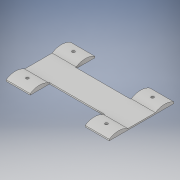
# Autodesk Inventor part: TapeMeasureBracketTop
Saved by Autodesk Inventor 2019 (Build 230136000, 136)
## iProperties
Created: 2018-11-07
Part Number: TapeMeasureBracketTop
Material: Generic
Document SubType Name: Modeling
Designer: Ashley
Density: 1 g/cm^3
Appearance: Default
Author: Ashley
Autodesk Inventor part; units mm, degrees
ref_plane "YZ Plane" through (0, 0, 0) normal (1, 0, 0) x (0, 1, 0)
ref_plane "XZ Plane" through (0, 0, 0) normal (0, 1, 0) x (-1, 0, 0)
ref_plane "XY Plane" through (0, 0, 0) normal (0, 0, 1) x (1, 0, 0)
sketch "Main Base Sketch" plane through (0, 0, 0) normal (0, 1, 0) x (-1, 0, 0)
  line L0 (75, -47) -> (75, 47)
  line L1 (-75, 47) -> (-75, -47)
  line L2 (-75, -47) -> (75, 47) construction
  line L3 (75, -47) -> (-75, 47) construction
  line L4 (-40, -47) -> (-40, -19)
  line L5 (-40, -19) -> (40, -19)
  line L6 (40, -19) -> (40, -47)
  line L7 (40, 19) -> (40, 47)
  line L8 (-40, 19) -> (40, 19)
  line L9 (-40, 47) -> (-40, 19)
  line L10 (75, 47) -> (40, 47)
  line L11 (-40, 47) -> (-75, 47)
  line L12 (-75, -47) -> (-40, -47)
  line L13 (40, -47) -> (75, -47)
  point P0 (0, 0)
  point P1 (0, 0)
  dimension "d0" = 94
  dimension "d1" = 35
  dimension "d2" = 35
  dimension "d3" = 80
  dimension "d4" = 150
  dimension "d5" = 28
  dimension "d6" = 94
  dimension "d8" = 80
  dimension "d9" = 28
  dimension "d27" = 28
  dimension "d28" = 38
  dimension "d37" = 0
  constraints: 28 end point, 6 parallel, 5 perpendicular, 2 horizontal, 2 midpoint
  measures "d0" distance of L0.start L0.end
  measures "d1" distance between parallel lines of L6 L0
  measures "d2" distance between parallel lines of L1 L4
  measures "d3" distance of L4.end L5.end
  measures "d4" distance between parallel lines of L1 L0
  measures "d5" distance of L5.end L6.end
  measures "d6" distance of L1.start L1.end
  measures "d8" distance of L8.start L7.start
  measures "d9" distance of L9.start L8.start
  measures "d27" distance of L7.start L7.end
  measures "d28" distance between parallel lines of L5 L8
  measures "d37" distance of point (0, 0) point (0, 0)
extrude "Main Base Extrusion" add sketch "Main Base Sketch" along normal blind 6
sketch "Middle Cut Sketch" plane through (0, 6, 0) normal (0, 1, 0) x (1, 0, 0)
  line L0 (-75, 47) -> (-75, -47) projected
  line L1 (75, 19) -> (-75, 19)
  line L2 (-75, 19) -> (-75, -19)
  line L3 (-75, -19) -> (75, -19)
  line L4 (75, -19) -> (75, 19)
  line L5 (-40, -19) -> (40, -19) projected
  line L6 (75, -47) -> (75, 47) projected
  line L7 (40, 19) -> (-40, 19) projected
  point P0 (0, 0)
  dimension "d18" = 0
  dimension "d19" = 0
  dimension "d34" = 0
  constraints: 8 end point, 2 parallel, 1 horizontal, 1 perpendicular, 1 point on line
  measures "d18" distance between parallel lines of L5 L3
  measures "d19" distance between parallel lines of L6 L4
  measures "d34" distance between parallel lines of L7 L1
extrude "Middle Cut" cut sketch "Middle Cut Sketch" against normal blind 4
sketch "Arc Sketch" plane through (75, 0, 47) normal (1, 0, 0) x (0, 0, -1)
  line L0 (27, 9.4354) -> (27, -6.3008)
  line L1 (13.5, 8.8022) -> (13.5, -9.7521)
  line L2 (-4.6363, 2) -> (37.5698, 2)
  line L3 (94, 0) -> (0, 0) projected
  arc A0 (27, 2) -> (0, 2) centre (13.5, -18.7813) ccw
  line L4 (0, 7.9962) -> (0, -1.9448)
  line L5 (0, 0) -> (0, 6) projected
  line L6 (0, 6) -> (0, 2)
  line L7 (28, 6) -> (0, 6) projected
  line L8 (0, 6) -> (28, 6)
  line L9 (28, 2) -> (28, 6) projected
  line L10 (28, 6) -> (28, 2)
  line L11 (28, 2) -> (27, 2)
  line L12 (94, 0) -> (94, 6) projected
  dimension "d25" = 13.5
  dimension "d26" = 2
  dimension "d29" = 13.5
  dimension "d30" = 27
  constraints: 16 end point, 3 point on line, 3 vertical, 2 collinear, 2 point on circle, 1 centre point, 1 horizontal, 1 perpendicular
  measures "d25" distance between parallel lines of L0 L1
  measures "d26" distance between parallel lines of L3 L2
  measures "d29" distance between parallel lines of L1 L4
  measures "d30" distance between parallel lines of L0 L4
extrude "Arc Cut" cut sketch "Arc Sketch" against normal through all contours L7 L9 L2 L0 | L0 A0 L7 | A0 L4 L7
mirror "Arc Mirror" about plane through (0, 0, 0) normal (0, 0, 1) of "Arc Cut"
sketch "Arc Holes Sketch" plane through (0, 0, 0) normal (0, -1, 0) x (1, 0, 0)
  circle A0 centre (57.5, 33.5) radius 2
  line L0 (75, -47) -> (75, 47) projected
  line L1 (40, 47) -> (40, 19) projected
  line L2 (40, 19) -> (-40, 19) projected
  line L3 (75, 47) -> (40, 47) projected
  line L4 (104.495, 0) -> (-129.4816, 0)
  line L5 (0, -57.7002) -> (0, 85.929)
  circle A1 centre (57.5, -33.5) radius 2
  circle A2 centre (-57.5, 33.5) radius 2
  circle A3 centre (-57.5, -33.5) radius 2
  point P0 (0, 0)
  dimension "d38" = 4
  dimension "d39" = 17.5
  dimension "d40" = 17.5
  dimension "d41" = 14.5
  dimension "d42" = 13.5
  constraints: 4 centre point, 4 end point, 3 symmetric about line, 1 horizontal, 1 vertical, 3 other
  measures "d38" diameter of A0
  measures "d39" distance from line of L0 A0.centre
  measures "d40" distance from line of A0.centre L1
  measures "d41" distance from line of A0.centre L2
  measures "d42" distance from line of L3 A0.centre
extrude "Arc Holes Cut" cut sketch "Arc Holes Sketch" against normal through all contours A0 | A1 | A2 | A3
body "Solid1"
